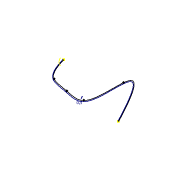
# Autodesk Inventor part: Fiber
Saved by Autodesk Inventor 2022.5 (Build 265521000, 521)
## iProperties
Created: 2024-03-12
Part Number: Fiber
Material: Generic
Document SubType Name: Modeling
Designer: wanghaoran
Density: 1 g/cm^3
Appearance: Default
Author: wanghaoran
Autodesk Inventor part; units mm, degrees
ref_plane "YZ Plane" through (0, 0, 0) normal (1, 0, 0) x (0, 1, 0)
ref_plane "XZ Plane" through (0, 0, 0) normal (0, 1, 0) x (-1, 0, 0)
ref_plane "XY Plane" through (0, 0, 0) normal (0, 0, 1) x (1, 0, 0)
sketch "Sketch1" plane through (0, 0, 0) normal (1, 0, 0) x (0, 1, 0)
  arc A0 (46.2493, 31.9968) -> (42.4397, 31.9409) centre (44.3714, 30.1371) ccw projected
  spline S0 degree 4 poles (0, 0) (19.619, -12.8758) (7.8139, 28.6781) (30.6578, 20.9092) (39.6678, 42.3298) (44.3714, 30.1371) knots 0 0 0 0 0 0.53761 1 1 1 1 1
  line L0 (45.3044, 30.4971) -> (44.3714, 30.1371)
  line L1 (0.5487, 0.836) -> (0, 0)
  spline S1 degree 5 poles (0.5487, 0.836) (1.6077, 0.1417) (2.6901, -0.5209) (3.8007, -1.1274) (5.5877, -1.9877) (7.4947, -2.5034) (8.1894, -2.6306) (9.3823, -2.6863) (10.5086, -2.3255) (10.9278, -2.0989) (11.7261, -1.4648) (12.3213, -0.6353) (12.5921, -0.16) (13.125, 0.941) (13.5225, 2.0989) (13.7172, 2.7467) (14.0873, 4.1255) (14.3991, 5.5184) (14.5541, 6.253) (14.8593, 7.7399) (15.1641, 9.227) (15.3223, 9.9777) (15.6496, 11.4536) (16.0216, 12.9189) (16.219, 13.6369) (16.6372, 15.0248) (17.1337, 16.3866) (17.3962, 17.0409) (17.9532, 18.295) (18.6051, 19.5023) (18.9455, 20.0764) (19.6602, 21.173) (20.4609, 22.2083) (20.8731, 22.7002) (21.7235, 23.6445) (22.6293, 24.536) (23.0883, 24.9663) (24.0208, 25.8111) (24.9743, 26.632) (25.454, 27.0389) (26.4193, 27.8505) (27.3877, 28.6585) (27.873, 29.0637) (28.8391, 29.8726) (29.8032, 30.684) (30.2832, 31.0888) (31.2277, 31.8853) (32.1764, 32.6768) (32.645, 33.0636) (33.5582, 33.8036) (34.4939, 34.5151) (34.9533, 34.8487) (35.8561, 35.4644) (36.8123, 35.9933) (37.2856, 36.2205) (38.2775, 36.5946) (39.3282, 36.7295) (39.868, 36.7161) (41.0094, 36.4779) (42.0031, 35.8562) (42.4708, 35.4344) (43.4825, 34.2959) (44.2381, 32.965) (44.6291, 32.1597) (44.9818, 31.3331) (45.3044, 30.4971) knots 0 0 0 0 0 0 0.089232 0.089232 0.089232 0.138804 0.138804 0.138804 0.171575 0.171575 0.171575 0.209973 0.209973 0.209973 0.257618 0.257618 0.257618 0.310504 0.310504 0.310504 0.364546 0.364546 0.364546 0.416986 0.416986 0.416986 0.466611 0.466611 0.466611 0.51357 0.51357 0.51357 0.558735 0.558735 0.558735 0.60305 0.60305 0.60305 0.64736 0.64736 0.64736 0.691892 0.691892 0.691892 0.736123 0.736123 0.736123 0.778925 0.778925 0.778925 0.818911 0.818911 0.818911 0.855816 0.855816 0.855816 0.893056 0.893056 0.893056 0.936846 0.936846 0.936846 1 1 1 1 1 1
  point P0 (14.5277, 2.0144)
  point P1 (19.5329, 19.0775)
  point P2 (28.6342, 28.3973)
  point P3 (37.7073, 35.284)
  dimension "d2" = 1
  constraints: 4 end point, 9 other
extrude "Extrusion1" add sketch "Sketch1" along normal blind 1
body "Solid1"
